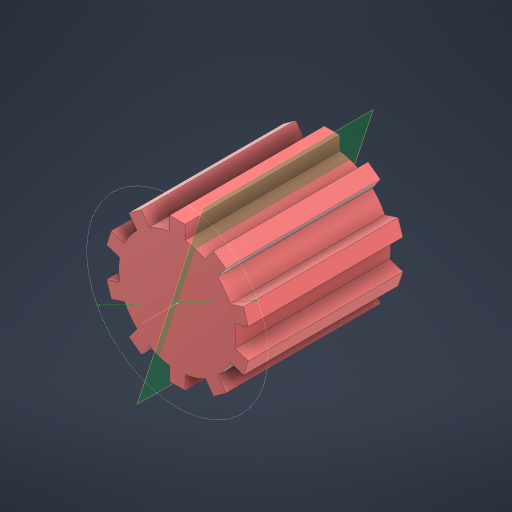
# Autodesk Inventor part: felga
Saved by Autodesk Inventor 2024 (Build 280153000, 153)
## iProperties
Created: 2024-05-21
Part Number: felga
Material: Generic
Document SubType Name: Modeling
Designer: Adam
Density: 1 g/cm^3
Appearance: Default
Author: Adam
Autodesk Inventor part; units mm, degrees
ref_plane "YZ Plane" through (0, 0, 0) normal (1, 0, 0) x (0, 1, 0)
ref_plane "XZ Plane" through (0, 0, 0) normal (0, 1, 0) x (-1, 0, 0)
ref_plane "XY Plane" through (0, 0, 0) normal (0, 0, 1) x (1, 0, 0)
sketch "Sketch1" plane through (0, 0, 0) normal (0, 0, 1) x (1, 0, 0)
  circle A0 centre (0, 0) radius 17 construction
  circle A1 centre (0, 0) radius 8.5
  line L0 (-1.4613, 13.5) -> (1.43, 13.5)
  line L1 (1.43, 13.5) -> (1.43, 10.9067)
  line L2 (-1.4613, 10.9025) -> (-1.4613, 13.5)
  line L3 (-6.7782, 11.7623) -> (-5.2539, 9.6642)
  line L4 (-9.1173, 10.0628) -> (-6.7782, 11.7623)
  line L5 (-7.5905, 7.9614) -> (-9.1173, 10.0628)
  line L6 (-12.3974, 5.5317) -> (-9.931, 4.7303)
  line L7 (-13.2908, 2.782) -> (-12.3974, 5.5317)
  line L8 (-10.8205, 1.9793) -> (-13.2908, 2.782)
  line L9 (-13.2812, -2.8117) -> (-10.8147, -2.0103)
  line L10 (-12.3877, -5.5615) -> (-13.2812, -2.8117)
  line L11 (-9.9173, -4.7588) -> (-12.3877, -5.5615)
  line L12 (-9.092, -10.0812) -> (-7.5677, -7.9831)
  line L13 (-6.7529, -11.7806) -> (-9.092, -10.0812)
  line L14 (-5.2261, -9.6792) -> (-6.7529, -11.7806)
  line L15 (-1.43, -13.5) -> (-1.43, -10.9067)
  line L16 (1.4613, -13.5) -> (-1.43, -13.5)
  line L17 (1.4613, -10.9025) -> (1.4613, -13.5)
  line L18 (6.7782, -11.7623) -> (5.2539, -9.6642)
  line L19 (9.1173, -10.0628) -> (6.7782, -11.7623)
  line L20 (7.5905, -7.9614) -> (9.1173, -10.0628)
  line L21 (12.3974, -5.5317) -> (9.931, -4.7303)
  line L22 (13.2908, -2.782) -> (12.3974, -5.5317)
  line L23 (10.8205, -1.9793) -> (13.2908, -2.782)
  line L24 (13.2812, 2.8117) -> (10.8147, 2.0103)
  line L25 (12.3877, 5.5615) -> (13.2812, 2.8117)
  line L26 (9.9173, 4.7588) -> (12.3877, 5.5615)
  line L27 (9.092, 10.0812) -> (7.5677, 7.9831)
  line L28 (6.7529, 11.7806) -> (9.092, 10.0812)
  line L29 (5.2261, 9.6792) -> (6.7529, 11.7806)
  arc A2 (-1.4613, 10.9025) -> (-5.2539, 9.6642) centre (0, 0) ccw construction
  arc A3 (-1.4613, 10.9025) -> (-5.2539, 9.6642) centre (0, 0) ccw
  arc A4 (-7.5905, 7.9614) -> (-9.931, 4.7303) centre (0, 0) ccw
  arc A5 (-7.5905, 7.9614) -> (-9.931, 4.7303) centre (0, 0) ccw construction
  arc A6 (-10.8205, 1.9793) -> (-10.8147, -2.0103) centre (0, 0) ccw
  arc A7 (-10.8205, 1.9793) -> (-10.8147, -2.0103) centre (0, 0) ccw construction
  arc A8 (-9.9173, -4.7588) -> (-7.5677, -7.9831) centre (0, 0) ccw
  arc A9 (-9.9173, -4.7588) -> (-7.5677, -7.9831) centre (0, 0) ccw construction
  arc A10 (5.2261, 9.6792) -> (1.43, 10.9067) centre (0, 0) ccw construction
  arc A11 (5.2261, 9.6792) -> (1.43, 10.9067) centre (0, 0) ccw
  arc A12 (10.8205, -1.9793) -> (10.8147, 2.0103) centre (0, 0) ccw
  arc A13 (10.8205, -1.9793) -> (10.8147, 2.0103) centre (0, 0) ccw construction
  arc A14 (7.5905, -7.9614) -> (9.931, -4.7303) centre (0, 0) ccw
  arc A15 (7.5905, -7.9614) -> (9.931, -4.7303) centre (0, 0) ccw construction
  arc A16 (-5.2261, -9.6792) -> (-1.43, -10.9067) centre (0, 0) ccw
  arc A17 (1.4613, -10.9025) -> (5.2539, -9.6642) centre (0, 0) ccw
  arc A18 (-5.2261, -9.6792) -> (-1.43, -10.9067) centre (0, 0) ccw construction
  arc A19 (1.4613, -10.9025) -> (5.2539, -9.6642) centre (0, 0) ccw construction
  arc A20 (9.9173, 4.7588) -> (7.5677, 7.9831) centre (0, 0) ccw
  dimension "d5" = 360
  dimension "d14" = 5
  dimension "d15" = 11
  dimension "d16" = 34
  dimension "d17" = 17
  dimension "d24" = 2.5933
  dimension "d25" = 2.8912
  constraints: 60 end point, 38 point on circle, 21 centre point, 5 coincident, 1 horizontal, 1 parallel, 1 perpendicular, 71 other
  measures "d14" distance edge to line of A1 L0
  measures "d15" radius of A2
  measures "d16" diameter of A0
  measures "d17" diameter of A1
  measures "d24" distance of L0.end L1.end
  measures "d25" distance of L0.start L0.end
extrude "Extrusion1" add sketch "Sketch1" along normal blind 29
sketch "Sketch2" plane through (0, 0, 29) normal (0, 0, 1) x (1, 0, 0)
  line L0 (-5.2539, 9.6642) -> (-6.7782, 11.7623) projected
  line L1 (-6.7782, 11.7623) -> (-9.1173, 10.0628) projected
  line L2 (-9.1173, 10.0628) -> (-7.5905, 7.9614) projected
  arc A0 (-7.5905, 7.9614) -> (-9.931, 4.7303) centre (0, 0) ccw projected
  line L3 (-9.931, 4.7303) -> (-12.3974, 5.5317) projected
  line L4 (-12.3974, 5.5317) -> (-13.2908, 2.782) projected
  line L5 (-13.2908, 2.782) -> (-10.8205, 1.9793) projected
  arc A1 (-10.8205, 1.9793) -> (-10.8147, -2.0103) centre (0, 0) ccw projected
  line L6 (-10.8147, -2.0103) -> (-13.2812, -2.8117) projected
  line L7 (-13.2812, -2.8117) -> (-12.3877, -5.5615) projected
  line L8 (-12.3877, -5.5615) -> (-9.9173, -4.7588) projected
  arc A2 (-9.9173, -4.7588) -> (-7.5677, -7.9831) centre (0, 0) ccw projected
  line L9 (-7.5677, -7.9831) -> (-9.092, -10.0812) projected
  line L10 (-9.092, -10.0812) -> (-6.7529, -11.7806) projected
  line L11 (-6.7529, -11.7806) -> (-5.2261, -9.6792) projected
  arc A3 (-5.2261, -9.6792) -> (-1.43, -10.9067) centre (0, 0) ccw projected
  line L12 (-1.43, -10.9067) -> (-1.43, -13.5) projected
  line L13 (-1.43, -13.5) -> (1.4613, -13.5) projected
  line L14 (1.4613, -13.5) -> (1.4613, -10.9025) projected
  arc A4 (1.4613, -10.9025) -> (5.2539, -9.6642) centre (0, 0) ccw projected
  line L15 (5.2539, -9.6642) -> (6.7782, -11.7623) projected
  line L16 (6.7782, -11.7623) -> (9.1173, -10.0628) projected
  line L17 (9.1173, -10.0628) -> (7.5905, -7.9614) projected
  arc A5 (7.5905, -7.9614) -> (9.931, -4.7303) centre (0, 0) ccw projected
  line L18 (9.931, -4.7303) -> (12.3974, -5.5317) projected
  line L19 (12.3974, -5.5317) -> (13.2908, -2.782) projected
  line L20 (13.2908, -2.782) -> (10.8205, -1.9793) projected
  arc A6 (10.8205, -1.9793) -> (10.8147, 2.0103) centre (0, 0) ccw projected
  line L21 (10.8147, 2.0103) -> (13.2812, 2.8117) projected
  line L22 (13.2812, 2.8117) -> (12.3877, 5.5615) projected
  line L23 (12.3877, 5.5615) -> (9.9173, 4.7588) projected
  arc A7 (9.9173, 4.7588) -> (7.5677, 7.9831) centre (0, 0) ccw projected
  line L24 (7.5677, 7.9831) -> (9.092, 10.0812) projected
  line L25 (9.092, 10.0812) -> (6.7529, 11.7806) projected
  line L26 (6.7529, 11.7806) -> (5.2261, 9.6792) projected
  arc A8 (5.2261, 9.6792) -> (1.43, 10.9067) centre (0, 0) ccw projected
  line L27 (1.43, 10.9067) -> (1.43, 13.5) projected
  line L28 (1.43, 13.5) -> (-1.4613, 13.5) projected
  line L29 (-1.4613, 13.5) -> (-1.4613, 10.9025) projected
  arc A9 (-1.4613, 10.9025) -> (-5.2539, 9.6642) centre (0, 0) ccw projected
  circle A10 centre (0, 0) radius 8.5 projected
  circle A11 centre (0, 0) radius 8.5
  constraints: 1 centre point, 1 coincident, 1 concentric
extrude "Extrusion2" add sketch "Sketch2" against normal blind 11 contours A10
sketch "Sketch3" plane through (0, 0, 18) normal (0, 0, -1) x (-1, 0, 0)
  arc A0 (1.3217, 0.7094) -> (0.5581, -1.3923) centre (0, 0) ccw
  line L0 (0.5581, -1.3923) -> (1.3217, 0.7094)
  circle A1 centre (0, 0) radius 2.5
  point P0 (0, 0)
  dimension "d11" = 5
  constraints: 2 centre point, 2 end point, 2 point on circle, 1 coincident, 1 other
  measures "d11" diameter of A1
extrude "Extrusion3" add sketch "Sketch3" along normal blind 9
ref_plane "Work Plane1" through (-0.4516, -1.3897, 0) normal (-0.9510565, 0.309017, 0) x (0, 0, 1)
sketch "Sketch4" plane through (-0.4516, -1.3897, 0) normal (-0.9510565, 0.309017, 0) x (0, 0, 1)
  line L0 (31.9338, 1.727) -> (-3.3978, 1.727) construction
  point P0 (0, 1.4613)
  constraints: 2 end point, 1 horizontal
ref_plane "Work Plane2" through (0, 0, 29) normal (0, 0, 1) x (1, 0, 0)
sketch "Sketch5" plane through (0, 0, 29) normal (0, 0, 1) x (1, 0, 0)
  circle A0 centre (0, 0) radius 17 construction
  dimension "d19" = 34
  constraints: 1 centre point, 1 coincident
  measures "d19" diameter of A0
body "Solid1"
